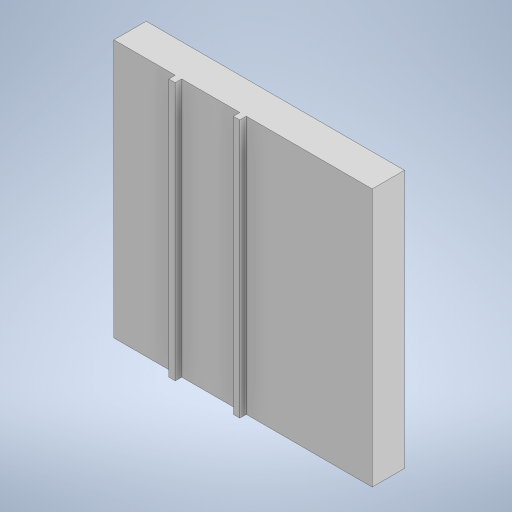
# Autodesk Inventor part: grating10
Saved by Autodesk Inventor 2023 (Build 270158000, 158)
## iProperties
Created: 2022-05-08
Part Number: grating10
Material: Generisch
Document SubType Name: Sheet Metal
Designer: t1mst
Density: 1 g/cm^3
Sheet Metal Rule: Standard_mm
Appearance: Vorgabe
Author: t1mst
Autodesk Inventor part; units mm, degrees
ref_plane "YZ Plane" through (0, 0, 0) normal (1, 0, 0) x (0, 1, 0)
ref_plane "XZ Plane" through (0, 0, 0) normal (0, 1, 0) x (-1, 0, 0)
ref_plane "XY Plane" through (0, 0, 0) normal (0, 0, 1) x (1, 0, 0)
sketch "Skizze1" plane through (0, 0, 0) normal (0, 0, 1) x (1, 0, 0)
  line L0 (0, 0) -> (0, 40)
  line L1 (0, 40) -> (40, 40)
  line L2 (40, 40) -> (40, 0)
  line L3 (40, 0) -> (0, 0)
  dimension "d0" = 40
  dimension "d1" = 40
  dimension "d2" = 40
  constraints: 8 end point, 2 vertical, 1 horizontal
  measures "d0" distance of L0.start L0.end
  measures "d1" distance of L0.end L1.end
  measures "d2" distance of L1.end L2.end
extrude "Extrusion1" add sketch "Skizze1" along normal blind 5
sketch "Skizze2" plane through (0, 0, 5) normal (0, 0, 1) x (1, 0, 0)
  line L0 (10.5001, 40) -> (10.5001, 0)
  line L1 (10.5001, 40) -> (9.5001, 40)
  line L2 (9.5001, 40) -> (9.5001, 0)
  line L3 (0, 0) -> (40, 0) projected
  line L4 (20.5001, 40) -> (20.5001, 0)
  line L5 (9.5001, 40) -> (10.5001, 40)
  line L6 (40, 40) -> (0, 40) projected
  line L7 (9.5001, 0) -> (10.5001, 0)
  dimension "d5" = 40
  dimension "d6" = 1
  constraints: 12 end point, 2 perpendicular, 2 point on line, 1 collinear, 1 horizontal, 1 vertical
  measures "d5" distance of L0.start L0.end
  measures "d6" distance of L0.start L1.end
extrude "Extrusion2" add sketch "Skizze2" along normal blind 1 contours L0 L3 L2 L1
sketch "Skizze3" plane through (0, 0, 5) normal (0, 0, 1) x (1, 0, 0)
  line L0 (20.5001, 40) -> (20.5001, 0)
  line L1 (20.5001, 40) -> (19.5001, 40)
  line L2 (40, 40) -> (10.5001, 40) projected
  line L3 (19.5001, 40) -> (19.5001, 0)
  line L4 (19.5001, 0) -> (20.5001, 0)
  line L5 (10.5001, 0) -> (40, 0) projected
  line L6 (19.5001, 40) -> (20.5001, 40)
  point P0 (0, 0)
  dimension "d11" = 40
  dimension "d12" = 1
  dimension "d13" = 40
  constraints: 10 end point, 2 collinear, 1 point on line
  measures "d11" distance of L0.start L0.end
  measures "d12" distance of L0.start L1.end
  measures "d13" distance of L1.end L3.end
extrude "Extrusion3" add sketch "Skizze3" along normal blind 1
equation "\"Biegeradius\" = Stärke"
equation "\"BreiteBiegungsfreistellung\" = Stärke"
equation "\"TiefeBiegungsfreistellung\" = 0.5 * Stärke"
equation "\"GrößeEckenfreistellung\" = 4 * Stärke"
equation "\"MinimalRest\" = 2 * Stärke"
equation "\"Übergangsradius\" = Biegeradius"
equation "\"JacobiRadiusGröße\" = Biegeradius"
equation "\"Abstandsgröße\" = Stärke"
equation "\"Stärke\" = 0.5"
